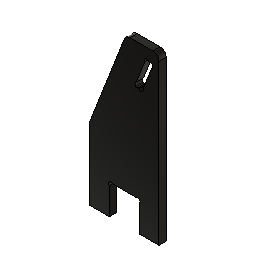
CameraTowerRight v2 (Autodesk Fusion 360 design; units mm, degrees)
Autodesk Fusion 360 part; units mm, degrees
sketch "Sketch1" plane through (0, 0, 0) normal (0, 1, 0) x (1, 0, 0)
  line L0 (46, -110) -> (0, -110)
  line L1 (0, -110) -> (0, 0)
  line L2 (13, 0) -> (13, -17.8787)
  line L3 (15.1213, -20) -> (30.8787, -20)
  line L4 (33, -17.8787) -> (33, 0)
  line L5 (0, 0) -> (13, 0)
  line L6 (33, 0) -> (46, 0)
  line L7 (13, 0) -> (33, 0) construction
  line L8 (30.1388, -84.5498) -> (37.3876, -103.1899) construction
  line L9 (37.3876, -103.1899) -> (41.8612, -101.4502) construction
  line L10 (41.8612, -101.4502) -> (34.6124, -82.8101) construction
  line L11 (34.6124, -82.8101) -> (30.1388, -84.5498) construction
  line L12 (37.3876, -103.1899) -> (34.6124, -82.8101) construction
  line L13 (37.3876, -103.1899) -> (37.9917, -101.817) construction
  line L14 (41.8612, -101.4502) -> (40.4882, -100.8461) construction
  line L15 (30.1388, -84.5498) -> (31.5118, -85.1539) construction
  line L16 (34.6124, -82.8101) -> (34.0083, -84.183) construction
  line L17 (39.3646, -102.4211) -> (39.8841, -102.2191)
  line L18 (36.6187, -101.2128) -> (30.9076, -86.5269)
  line L19 (32.1159, -83.7809) -> (32.6354, -83.5789)
  line L20 (35.3813, -84.7872) -> (41.0924, -99.4731)
  arc A0 (39.3646, -102.4211) -> (36.6187, -101.2128) centre (37.9917, -101.817) ccw construction
  arc A1 (37.3876, -103.1899) -> (39.3646, -102.4211) centre (37.9917, -101.817) ccw
  arc A2 (36.6187, -101.2128) -> (37.3876, -103.1899) centre (37.9917, -101.817) ccw
  arc A3 (41.0924, -99.4731) -> (39.8841, -102.2191) centre (40.4882, -100.8461) ccw construction
  arc A4 (39.8841, -102.2191) -> (41.8612, -101.4502) centre (40.4882, -100.8461) ccw
  arc A5 (41.8612, -101.4502) -> (41.0924, -99.4731) centre (40.4882, -100.8461) ccw
  arc A6 (30.9076, -86.5269) -> (32.1159, -83.7809) centre (31.5118, -85.1539) ccw construction
  arc A7 (32.1159, -83.7809) -> (30.1388, -84.5498) centre (31.5118, -85.1539) ccw
  arc A8 (30.1388, -84.5498) -> (30.9076, -86.5269) centre (31.5118, -85.1539) ccw
  arc A9 (32.6354, -83.5789) -> (35.3813, -84.7872) centre (34.0083, -84.183) ccw construction
  arc A10 (34.6124, -82.8101) -> (32.6354, -83.5789) centre (34.0083, -84.183) ccw
  arc A11 (35.3813, -84.7872) -> (34.6124, -82.8101) centre (34.0083, -84.183) ccw
  line L21 (38.2368, -92.1301) -> (61.537, -83.0692) construction
  line L22 (57.0065, -71.4191) -> (66.0675, -94.7193) construction
  line L23 (66.0675, -94.7193) -> (44.7444, -103.0114) construction
  line L24 (57.0065, -71.4191) -> (35.6834, -79.7112) construction
  line L25 (32.6354, -83.5789) -> (34.6124, -82.8101) construction
  line L26 (34.6124, -82.8101) -> (34.4752, -82.4571) construction
  line L27 (35.6834, -79.7112) -> (46, -75.6993) construction
  line L28 (39.8841, -102.2191) -> (41.8612, -101.4502) construction
  line L29 (41.8612, -101.4502) -> (41.9984, -101.8032) construction
  line L30 (44.7444, -103.0114) -> (46, -102.5231) construction
  line L31 (46, 0) -> (46, -75.6993)
  line L32 (46, -102.5231) -> (46, -110)
  line L33 (46, -89.1112) -> (46, -102.5231)
  line L34 (42.7673, -103.7802) -> (43.3714, -102.4073) construction
  arc A12 (41.9984, -101.8032) -> (42.7673, -103.7802) centre (43.3714, -102.4073) ccw construction
  arc A13 (44.7444, -103.0114) -> (41.9984, -101.8032) centre (43.3714, -102.4073) ccw construction
  arc A14 (42.7673, -103.7802) -> (44.7444, -103.0114) centre (43.3714, -102.4073) ccw construction
  line L35 (41.9984, -101.8032) -> (42.7673, -103.7802) construction
  line L36 (44.7444, -103.0114) -> (42.7673, -103.7802) construction
  line L37 (42.7673, -103.7802) -> (44.7444, -103.0114) construction
  line L38 (46, -75.6993) -> (46, -89.1112)
  line L39 (33.7063, -80.4801) -> (35.0793, -81.0842) construction
  arc A15 (35.6834, -79.7112) -> (34.4752, -82.4571) centre (35.0793, -81.0842) ccw construction
  arc A16 (34.4752, -82.4571) -> (35.6834, -79.7112) centre (35.0793, -81.0842) ccw construction
  line L40 (34.4752, -82.4571) -> (33.7063, -80.4801) construction
  line L41 (35.6834, -79.7112) -> (33.7063, -80.4801) construction
  line L42 (33.7063, -80.4801) -> (35.6834, -79.7112) construction
  line L43 (13, -20) -> (14.0607, -18.9393) construction
  line L44 (33, -20) -> (31.9393, -18.9393) construction
  arc A17 (13, -17.8787) -> (15.1213, -20) centre (14.0607, -18.9393) ccw
  arc A18 (15.1213, -20) -> (13, -17.8787) centre (14.0607, -18.9393) ccw construction
  arc A19 (30.8787, -20) -> (33, -17.8787) centre (31.9393, -18.9393) ccw
  arc A20 (33, -17.8787) -> (30.8787, -20) centre (31.9393, -18.9393) ccw construction
  line L45 (13, -17.8787) -> (13, -20) construction
  line L46 (13, -20) -> (15.1213, -20) construction
  line L47 (30.8787, -20) -> (33, -20) construction
  line L48 (33, -20) -> (33, -17.8787) construction
  point P0 (36, -93)
  point P1 (38.2368, -92.1301)
  point P2 (61.537, -83.0692)
  dimension "d2" = 110
  dimension "d3" = 20
  dimension "d4" = 20
  dimension "d5" = 13
  dimension "d6" = 46
  dimension "d7" = 13
  dimension "d15" = 20
  dimension "d16" = 4.8
  dimension "d17" = 21.25
  dimension "d18" = 1.5
  dimension "d19" = 1.5
  dimension "d20" = 45
  dimension "d21" = 45
  dimension "d22" = 1.5
  dimension "d23" = 1.5
  dimension "d24" = 45
  dimension "d25" = 45
  dimension "d26" = 25
  dimension "d29" = 84.1301
  dimension "d30" = 25.2368
  dimension "d31" = 25
  dimension "d32" = 36
  dimension "d33" = 17
  dimension "d34" = 1.5
  dimension "d35" = 45
  dimension "d36" = 1.5
  dimension "d37" = 45
  dimension "d48" = 1.5
  dimension "d49" = 1.5
  dimension "d50" = 45
  dimension "d51" = 45
  constraint horizontal L5
  constraint vertical L31
  constraint horizontal L0
  constraint vertical L1
  constraint coincident L1.end L5.start
  constraint perpendicular L2 L5
  constraint perpendicular L2 L3
  constraint coincident L4.end L5
  constraint perpendicular L4 L5
  constraint perpendicular L8 L9
  constraint perpendicular L9 L10
  constraint perpendicular L10 L11
  constraint midpoint L12 P0
  constraint coincident L15.end A6.centre
  constraint coincident L16.end A9.centre
  constraint coincident L13.end A0.centre
  constraint coincident L14.end A3.centre
  constraint coincident L9 L17.start
  constraint coincident L9 L17.end
  constraint coincident L8 L18.start
  constraint coincident L8 L18.end
  constraint coincident L11 L19.start
  constraint coincident L11 L19.end
  constraint coincident L10 L20.start
  constraint coincident L10 L20.end
  constraint concentric A0 A1
  constraint concentric A0 A2
  constraint concentric A3 A4
  constraint concentric A3 A5
  constraint concentric A6 A7
  constraint concentric A6 A8
  constraint concentric A9 A10
  constraint concentric A9 A11
  constraint midpoint L20 P1
  constraint coincident P1 L21.start
  constraint perpendicular L20 L21
  constraint midpoint L22 P2
  constraint coincident P2 L21.end
  constraint perpendicular L21 L22
  constraint perpendicular L22 L23
  constraint perpendicular L22 L24
  constraint perpendicular L24 L26
  constraint coincident L24 L27.end
  constraint perpendicular L23 L29
  constraint coincident L30.end L31
  constraint coincident L23 L30.end
  constraint coincident L21 L33.start
  constraint perpendicular L0 L32
  constraint coincident L34.end A12.centre
  constraint concentric A12 A13
  constraint concentric A12 A14
  constraint perpendicular L23 L35
  constraint perpendicular L22 L36
  constraint vertical L38
  constraint coincident L39.end A15.centre
  constraint coincident L39.start A15
  constraint concentric A15 A16
  constraint perpendicular L24 L40
  constraint perpendicular L22 L41
  constraint coincident L43.end A17.centre
  constraint coincident L43.start A17
  constraint coincident L44.end A19.centre
  constraint coincident L44.start A19
  constraint concentric A17 A18
  constraint concentric A19 A20
  constraint perpendicular L5 L45
  constraint perpendicular L2 L46
  constraint perpendicular L2 L47
  constraint perpendicular L5 L48
  measures "d2" distance of L1.end L0.end
  measures "d3" distance of L2.start L43.start
  measures "d4" distance of L43.start L44.start
  measures "d5" distance of L1 L2
  measures "d6" distance of L1 L31
  measures "d7" distance of L6.end L4.end
  measures "d15" distance of L8.start L8.end
  measures "d16" distance of L8.end L9.end
  measures "d17" angle of L0 L9
  measures "d18" distance of L8.end L13.end
  measures "d19" distance of L9.end L14.end
  measures "d20" angle of L9 L13
  measures "d21" angle of L9 L14
  measures "d22" distance of L8.start L15.end
  measures "d23" distance of L10.end L16.end
  measures "d24" angle of L11 L15
  measures "d25" angle of L11 L16
  measures "d26" distance of P1 P2
  measures "d31" distance of L22.start L22.end
  measures "d32" distance of L1 P0
  measures "d33" distance of L0 P0
  measures "d34" distance of L34.start L34.end
  measures "d35" angle of L30 L34
  measures "d36" distance of L39.start L39.end
  measures "d37" angle of L24 L39
  measures "d48" distance of L43.start L43.end
  measures "d49" distance of L44.start L44.end
  measures "d50" angle of L3 L43
  measures "d51" angle of L3 L44
extrude "Extrude1" add sketch "Sketch1" along normal blind 4.8
fillet "Fillet1" radius 4 2 edges at (0, 2.4, 110) (46, 2.4, 110)
sketch "Sketch2" plane through (0, 0, 0) normal (0, 0, -1) x (1, 0, 0)
  line L0 (13, 0) -> (0, 0)
  line L1 (0, 0) -> (0, -4.8)
  line L2 (0, -4.8) -> (13, -4.8)
  line L3 (13, -4.8) -> (13, 0)
  line L4 (46, 0) -> (33, 0)
  line L5 (33, 0) -> (33, -4.8)
  line L6 (33, -4.8) -> (46, -4.8)
  line L7 (46, -4.8) -> (46, 0)
  line L8 (0, 0) -> (13, -4.8) construction
  line L9 (33, 0) -> (46, -4.8) construction
  circle A0 centre (6.5, -2.4) radius 1.5
  circle A1 centre (39.5, -2.4) radius 1.5
  point P0 (6.5, -2.4)
  point P1 (39.5, -2.4)
  dimension "d52" = 3
  dimension "d53" = 3
  constraint coincident L0.end L1.start
  constraint coincident L2.end L3.start
  constraint coincident L4.end L5.start
  constraint coincident L6.end L7.start
  constraint midpoint L8 P0
  constraint midpoint L9 P1
  constraint coincident P0 A0.centre
  constraint coincident P1 A1.centre
  measures "d52" diameter of A0
  measures "d53" diameter of A1
extrude "Extrude2" cut sketch "Sketch2" against normal blind 8 contours A0 | A1
thread "Thread1" "ISO Metric profile 3.0 M3x0.5 6H" major diameter 3.086 minor diameter 2.529 pitch 0.5 angle 60 modelled right hand crest width 0.1368 on face at (7.9981, 2.4748, 5.3333) crest through (7.7645, 2.4, 0.125)
thread "Thread2" "ISO Metric profile 3.0 M3x0.5 6H" major diameter 3.086 minor diameter 2.529 pitch 0.5 angle 60 modelled right hand crest width 0.1368 on face at (39.9063, 0.9561, 5.3333) crest through (40.7645, 2.4, 0.125)
sketch "Sketch3" plane through (0, 0, 0) normal (0, -1, 0) x (1, 0, 0)
  arc A0 (39.3646, 102.4211) -> (36.6187, 101.2128) centre (37.9917, 101.817) ccw
  line L0 (39.3646, 102.4211) -> (39.8841, 102.2191)
  arc A1 (41.0924, 99.4731) -> (39.8841, 102.2191) centre (40.4882, 100.8461) ccw
  line L1 (41.0924, 99.4731) -> (35.3813, 84.7872)
  arc A2 (32.6354, 83.5789) -> (35.3813, 84.7872) centre (34.0083, 84.183) ccw
  line L2 (32.6354, 83.5789) -> (32.1159, 83.7809)
  arc A3 (30.9076, 86.5269) -> (32.1159, 83.7809) centre (31.5118, 85.1539) ccw
  line L3 (30.9076, 86.5269) -> (36.6187, 101.2128)
  arc A4 (46, 106) -> (42, 110) centre (42, 106) ccw
  line L4 (42, 110) -> (4, 110)
  arc A5 (4, 110) -> (0, 106) centre (4, 106) ccw
  line L5 (0, 106) -> (0, 0)
  line L6 (0, 0) -> (13, 0)
  line L7 (13, 0) -> (13, 17.8787)
  arc A6 (15.1213, 20) -> (13, 17.8787) centre (14.0607, 18.9393) ccw
  line L8 (15.1213, 20) -> (30.8787, 20)
  arc A7 (33, 17.8787) -> (30.8787, 20) centre (31.9393, 18.9393) ccw
  line L9 (33, 17.8787) -> (33, 0)
  line L10 (33, 0) -> (46, 0)
  line L11 (46, 0) -> (46, 106)
  line L12 (23.9416, 110) -> (0, 48.4344)
  line L13 (36.6187, 101.2128) -> (30.9076, 86.5269)
  dimension "d58" = 15
  constraint coincident L4 L12.start
  constraint coincident L5 L12.end
  constraint parallel L12 L13
  measures "d58" distance of L12 L13
extrude "Extrude3" cut sketch "Sketch3" against normal through all contours L4 A5 L5 L12
fillet "Fillet2" radius 4 2 edges at (23.9416, 2.4, 110) (0, 2.4, 48.4344)
